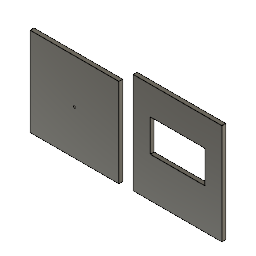
AssemblyPanels (Autodesk Fusion 360 design; units mm, degrees)
Autodesk Fusion 360 part; units mm, degrees
sketch "Sketch1" plane through (0, 0, 0) normal (0, 1, 0) x (1, 0, 0)
  line L0 (0, 0) -> (220, 0)
  line L1 (220, 0) -> (220, -220)
  line L2 (220, -220) -> (0, -220)
  line L3 (0, -220) -> (0, 0)
  circle A0 centre (110, -110) radius 2.4
  line L4 (255.3203, -2.6922) -> (475.3203, -2.6922)
  line L5 (475.3203, -2.6922) -> (475.3203, -252.6922)
  line L6 (475.3203, -252.6922) -> (255.3203, -252.6922)
  line L7 (255.3203, -252.6922) -> (255.3203, -2.6922)
  line L8 (297.8463, -102.6922) -> (297.8463, -182.6922)
  line L9 (297.8463, -102.6922) -> (432.8463, -102.6922)
  line L10 (297.8463, -182.6922) -> (432.8463, -182.6922)
  line L11 (432.8463, -182.6922) -> (432.8463, -102.6922)
  dimension "d1" = 220
  dimension "d2" = 220
  dimension "d3" = 4.8
  dimension "d4" = 250
  dimension "d5" = 220
  dimension "d10" = 135
  dimension "d12" = 80
  constraint horizontal L0
  constraint vertical L1
  constraint horizontal L2
  constraint vertical L3
  constraint coincident L0.start L3.end
  constraint horizontal L4
  constraint vertical L5
  constraint horizontal L6
  constraint vertical L7
  constraint perpendicular L8 L9
  constraint perpendicular L8 L10
  measures "d1" distance of L0.start L2.end
  measures "d2" distance of L1.end L2.end
  measures "d3" diameter of A0
  measures "d4" distance of L4.start L6.end
  measures "d5" distance of L5.end L6.end
  measures "d10" distance of L8.start L9.end
  measures "d12" distance of L9.end L10.end
extrude "Extrude1" add sketch "Sketch1" along normal blind 10 contours L0 L1 L2 L3 makes body 1
extrude "Extrude2" add sketch "Sketch1" along normal blind 10 separate body contours L4 L5 L6 L7 makes body 2
